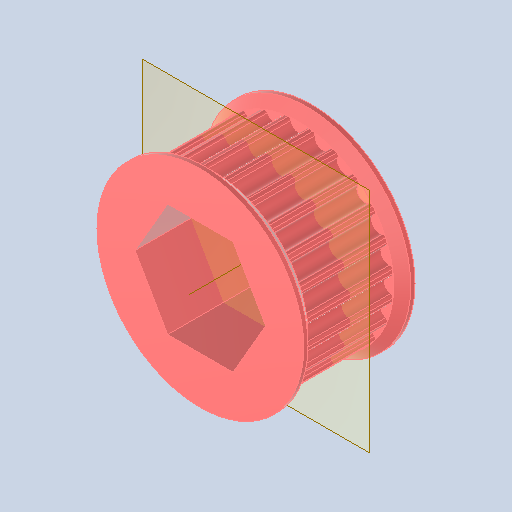
# Autodesk Inventor part: 24T_GT2_1_2_HexBore_9mm_wide_Flanged_Pulley
Saved by Autodesk Inventor 2022.3 (Build 263350000, 350)
## iProperties
RuleStatus: InUse
Created: 2020-06-08
Part Number: 24T_GT2_1_2_HexBore_9mm_wide_Flanged_Pulley
Material: ABS Plastic
Document SubType Name: Modeling
Designer: Bryce
Density: 1.06 g/cm^3
Appearance: Smooth - Red
Mass: 2.94962 g
Surface Area: 25.2365 cm^2
Volume: 2.78266 cm^3
Author: Bryce
Autodesk Inventor part; units mm, degrees
ref_plane "YZ Plane" through (0, 0, 0) normal (1, 0, 0) x (0, 1, 0)
ref_plane "XY Plane" through (0, 0, 0) normal (0, 0, 1) x (1, 0, 0)
sketch "Sketch1" plane through (0, 0, 0) normal (0, 1, 0) x (-1, 0, 0)
  circle A0 centre (0, 0) radius 18.5271
  dimension "d0" = 37.0542
  constraints: 1 centre point, 1 coincident
  measures "d0" diameter of A0
extrude "HTD Base" [suppressed]
sketch "Sketch3" plane through (0, 8, 0) normal (0, 1, 0) x (1, 0, 0)
  circle A0 centre (0, 0) radius 19.5271
  arc A1 (-1.5181, 18.4648) -> (1.5181, 18.4648) centre (0, 0) ccw construction
  line L0 (0, 18.5271) -> (0, 19.5271)
  point P0 (-1.9949, 18.4194)
  point P1 (-2.8404, 18.3081)
  point P2 (1.9949, 18.4194)
  dimension "d12" = 1
  constraints: 2 end point, 2 point on circle, 1 coincident, 1 line through centre, 1 vertical alignment, 2 other
  measures "d12" distance of L0.start L0.end
extrude "HTD Flange" [suppressed]
mirror "HTD Flanges" [suppressed]
chamfer "HTD Flange Chamfer" [suppressed]
sketch "Sketch6" plane through (0, 0, 0) normal (0, 1, 0) x (-1, 0, 0)
  circle A0 centre (0, 0) radius 11.0782
  dimension "d24" = 22.1563
  constraints: 1 centre point, 1 coincident
  measures "d24" diameter of A0
extrude "GT2 Base" add sketch "Sketch6" against normal mid plane 10
sketch "Sketch7" plane through (0, 0, 0) normal (0, 1, 0) x (-1, 0, 0)
  circle A0 centre (0, -10.8877) radius 0.923
  line L0 (0, -10.8877) -> (0, -11.0782) construction
  circle A1 centre (0, 0) radius 11.0782 construction
  dimension "d27" = 1.846
  dimension "d28" = 0.1905
  constraints: 2 end point, 2 vertical alignment, 1 centre point, 1 vertical, 1 other
  measures "d27" diameter of A0
  measures "d28" distance of L0.start L0.end
extrude "GT2 Base Tooth" cut sketch "Sketch7" against normal through all both and the other way through all
fillet "GT2 Base Tooth pt. 2" radius 0.299 2 edges at (0.9102, 0, -11.0407) (-0.9102, 0, -11.0407)
pattern_circular "GT2 Teeth" count 24 over 360 about axis through (0, -10, 0) along (0, 1, 0) of "GT2 Base Tooth", "GT2 Base Tooth pt. 2"
sketch "Sketch8" plane through (0, 5, 0) normal (0, 1, 0) x (1, 0, 0)
  circle A0 centre (0, 0) radius 12.0782
  arc A1 (-1.2427, 11.0082) -> (-1.6488, 10.9548) centre (0, 0) ccw construction
  line L0 (-1.446, 10.9834) -> (-1.5765, 11.9748) construction
  dimension "d35" = 1
  constraints: 2 end point, 2 point on circle, 1 coincident, 1 line through centre, 1 point on line, 4 other
  measures "d35" distance of L0.start L0.end
extrude "GT2 Flange" add sketch "Sketch8" along normal blind 1.5
mirror "GT2 Flanges" about plane through (0, 0, 0) normal (0, 1, 0) of "GT2 Flange"
chamfer "GT2 Flange Chamfer" distance 1 angle 45 2 edges at (-12.0782, 5, 0) (-12.0782, -5, 0)
sketch "Sketch4" plane through (0, 0, 0) normal (0, 1, 0) x (-1, 0, 0)
  line L0 (-3.8128, -6.604) -> (-7.6256, 0)
  line L1 (-7.6256, 0) -> (-3.8128, 6.604)
  line L2 (-3.8128, 6.604) -> (3.8128, 6.604)
  line L3 (3.8128, 6.604) -> (7.6256, 0)
  line L4 (7.6256, 0) -> (3.8128, -6.604)
  line L5 (3.8128, -6.604) -> (-3.8128, -6.604)
  point P0 (0, 0)
  point P1 (0, 0)
  dimension "d18" = 13.208
  constraints: 12 end point, 1 coincident, 1 horizontal, 13 other
  measures "d18" distance between parallel lines of L2 L5
extrude "Hex Bore" cut sketch "Sketch4" along normal through all both and the other way through all
sketch "Sketch5" plane through (0, 0, 0) normal (0, 1, 0) x (-1, 0, 0)
  circle A0 centre (0, 0) radius 6.604
  dimension "d21" = 13.208
  constraints: 1 centre point, 1 coincident
  measures "d21" diameter of A0
extrude "Circle Bore" [suppressed]
equation "\"d0\" = htd_od"
equation "\"d1\" = tooth_width"
equation "\"d12\" = flange_height"
equation "\"d13\" = flange_width"
equation "\"d15\" = flange_height"
equation "\"d24\" = gt2_od"
equation "\"d25\" = tooth_width"
equation "\"d28\" = 0.5 * gt2_pld"
equation "\"d35\" = flange_height"
equation "\"d36\" = flange_width"
equation "\"d38\" = flange_height"
equation "\"d18\" = bore_size"
equation "\"d21\" = bore_size"
equation "\"htd_pitch\" = 5"
equation "\"htd_pld\" = 0.5715"
equation "\"htd_od\" = htd_pd - 2 * htd_pld"
equation "\"tooth_width\" = 10"
equation "\"flange_width\" = 1.5"
equation "\"flange_height\" = 1"
equation "\"bore_size\" = 13.208"
equation "\"gt2_pitch\" = 3"
equation "\"gt2_pld\" = 0.381"
equation "\"gt2_od\" = gt2_pd - 2 * gt2_pld"
equation "\"htd_pd\" = 38.197186"
equation "\"gt2_pd\" = 22.918312"
body "Solid1"
